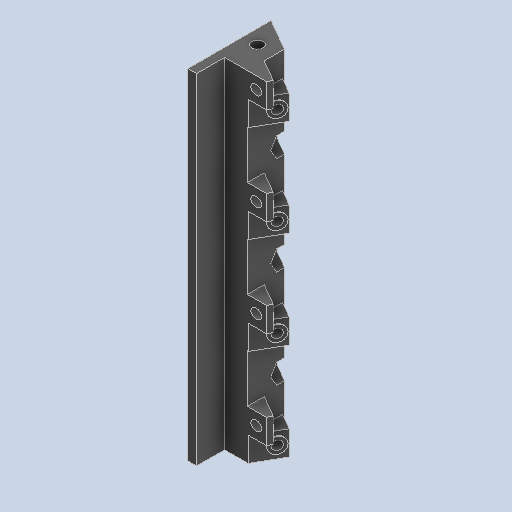
# Autodesk Inventor part: base_bearingpole_front
Saved by Autodesk Inventor 2024.1 (Build 281209000, 209)
## iProperties
Created: 2025-01-17
Part Number: base_bearingpole_front
Material: 一般
Document SubType Name: Modeling
Designer: hibik
Density: 1 g/cm^3
Appearance: 既定
Author: hibik
Autodesk Inventor part; units mm, degrees
ref_plane "YZ Plane" through (0, 0, 0) normal (1, 0, 0) x (0, 1, 0)
ref_plane "XZ Plane" through (0, 0, 0) normal (0, 1, 0) x (-1, 0, 0)
ref_plane "XY Plane" through (0, 0, 0) normal (0, 0, 1) x (1, 0, 0)
sketch "スケッチ1" plane through (0, 0, 0) normal (0, 1, 0) x (-1, 0, 0)
  line L0 (0, 0) -> (10, 0)
  line L1 (10, 0) -> (10, -23.7735)
  line L2 (0, 0) -> (0, -18) construction
  line L3 (0, -18) -> (10, -23.7735)
  line L4 (1, -18.5774) -> (1, 0)
  line L5 (-5, 0) -> (-5, -8)
  line L6 (0, -18) -> (-8.0801, -13.3349)
  line L7 (-8.0801, -13.3349) -> (-5, -8)
  line L8 (1, -12.8038) -> (-5.5801, -9.0048)
  line L9 (-1.25, -11.5048) -> (-3.75, -15.8349)
  line L10 (-5, -8) -> (1, -8)
  line L11 (-5.1471, -9.2548) -> (-4.4226, -8)
  line L12 (-1.25, -11.5048) -> (0.7735, -8)
  line L13 (-7.8301, -12.9019) -> (1, -18)
  line L14 (1, -8) -> (2, -8)
  line L15 (2, -8) -> (2, 0)
  line L16 (2, 0) -> (1, 0)
  line L17 (1, 0) -> (1, -8)
  point P0 (-3.5, -15.4019)
  dimension "d0" = 18
  dimension "d1" = 10
  dimension "d2" = 60
  dimension "d3" = 1
  dimension "d6" = 8
  dimension "d7" = 5
  dimension "d8" = 5
  dimension "d9" = 5
  dimension "d10" = 0.5
  dimension "d35" = 0.5
  dimension "d38" = 1
  constraints: 36 end point, 14 point on line, 5 perpendicular, 4 parallel, 4 vertical, 2 collinear, 2 horizontal
  measures "d0" distance of L0.start L2.end
  measures "d1" distance of L0.start L0.end
  measures "d2" angle of L2 L3
  measures "d3" distance between parallel lines of L2 L4
  measures "d6" distance of L5.start L5.end
  measures "d7" distance between parallel lines of L2 L5
  measures "d8" distance between parallel lines of L6 L8
  measures "d9" distance between parallel lines of L7 L9
  measures "d10" distance between parallel lines of L7 L11
  measures "d35" distance between parallel lines of L6 L13
  measures "d38" distance of L10.end L14.end
extrude "押し出し1" add sketch "スケッチ1" along normal blind 97 contours L0 L1 L3 L4 L14 L15
extrude "押し出し2" add sketch "スケッチ1" along normal blind 7 contours L4 L8 L12 L10 | L4 L13 L9 L8
sketch "スケッチ2" plane through (0, 7, 0) normal (0, 1, 0) x (1, 0, 0)
  line L0 (-1, 12.8038) -> (5.5801, 9.0048) projected
  line L1 (5.1471, 9.2548) -> (4.4226, 8) projected
  line L2 (5, 8) -> (-1, 8) projected
  line L3 (-1, 8) -> (-1, 18) projected
  point P0 (0, 0)
  point P1 (-1, 18.5774)
extrude "押し出し3" add sketch "スケッチ2" along normal blind 7
sketch "スケッチ3" plane through (3.75, 0, -15.8349) normal (0.8660254, 0, 0.5) x (0.5, 0, -0.8660254)
  circle A0 centre (-3, 3.5) radius 3
  line L0 (0, 0) -> (0, 7)
  circle A1 centre (-3, 3.5) radius 1.3
  line L1 (-0.5, 0) -> (-0.5, 7) projected
  point P0 (-15.5885, 0)
  point P1 (0, 3.5)
  dimension "d15" = 6
  dimension "d16" = 2.6
  dimension "d36" = 0.5
  constraints: 3 horizontal alignment, 2 centre point, 2 end point, 1 coincident, 1 midpoint, 1 tangent
  measures "d15" diameter of A0
  measures "d16" diameter of A1
  measures "d36" distance between parallel lines of L0 L1
extrude "押し出し4" cut sketch "スケッチ3" against normal blind 5 contours A1
sketch "スケッチ4" plane through (-1, 7, -12.8038) normal (0.5, 0, -0.8660254) x (-0.8660254, 0, -0.5)
  circle A0 centre (-4.5981, 3.5) radius 3
  line L0 (-7.5981, 0) -> (-7.5981, 7)
  circle A1 centre (-4.5981, 3.5) radius 1.35
  line L1 (-7.0981, 0) -> (-7.0981, 7) projected
  point P0 (-7.2679, -7)
  point P1 (-7.5981, 3.5)
  dimension "d19" = 6
  dimension "d20" = 2.7
  dimension "d37" = 0.5
  constraints: 3 horizontal alignment, 2 centre point, 2 end point, 1 coincident, 1 midpoint, 1 tangent
  measures "d19" diameter of A0
  measures "d20" diameter of A1
  measures "d37" distance between parallel lines of L1 L0
extrude "押し出し5" cut sketch "スケッチ4" against normal up to surface contours A1 surface through (-2, 0, -8) normal (0, 0, 1)
sketch "スケッチ5" plane through (3.75, 0, -15.8349) normal (0.8660254, 0, 0.5) x (0.5, 0, -0.8660254)
  circle A0 centre (-3, 3.5) radius 1.3 projected
  line L0 (-9.047, 0) -> (-0.5, 0) projected
  line L1 (-5, 7) -> (-0.5, 7) projected
  line L2 (-9.047, 7) -> (-5, 7) projected
  line L3 (-9.047, 0) -> (-9.047, 7) projected
  circle A1 centre (-3, 3.5) radius 2.25
  line L4 (-0.5, 0) -> (-0.5, 7) projected
  point P0 (-15.5885, 0)
  dimension "d26" = 4.5
  constraints: 1 centre point, 1 coincident
  measures "d26" diameter of A1
extrude "押し出し6" add sketch "スケッチ5" along normal blind 0.2 contours A1
sketch "スケッチ6" plane through (-1, 7, -12.8038) normal (0.5, 0, -0.8660254) x (-0.8660254, 0, -0.5)
  circle A0 centre (-4.5981, 3.5) radius 1.35 projected
  line L0 (-7.0981, 0) -> (-2.5981, 0) projected
  line L1 (0, 0) -> (-2.5981, 0) projected
  line L2 (0, 7) -> (0, 0) projected
  line L3 (-7.0981, 7) -> (0, 7) projected
  line L4 (-7.0981, 0) -> (-7.0981, 7) projected
  circle A1 centre (-4.5981, 3.5) radius 2.25
  point P0 (-7.2679, -7)
  dimension "d29" = 4.5
  constraints: 1 centre point, 1 coincident
  measures "d29" diameter of A1
extrude "押し出し7" add sketch "スケッチ6" along normal blind 0.2 contours A1
pattern_linear "矩形状パターン2" count 4 spacing 27.6667 along (0, 1, 0) of "押し出し2", "押し出し3", "押し出し4", "押し出し5", "押し出し6", "押し出し7"
sketch "スケッチ7" plane through (0, 97, 0) normal (0, 1, 0) x (1, 0, 0)
  line L0 (-8.85, 6.6454) -> (-6, 8.2909)
  line L1 (-6, 8.2909) -> (-3.15, 6.6454)
  line L2 (-3.15, 6.6454) -> (-3.15, 3.3546)
  line L3 (-3.15, 3.3546) -> (-6, 1.7091)
  line L4 (-6, 1.7091) -> (-8.85, 3.3546)
  line L5 (-8.85, 3.3546) -> (-8.85, 6.6454)
  line L6 (-8.85, 14.2184) -> (-8.85, 17.5093)
  line L7 (-8.85, 17.5093) -> (-6, 19.1547)
  line L8 (-6, 19.1547) -> (-3.15, 17.5093)
  line L9 (-3.15, 17.5093) -> (-3.15, 14.2184)
  line L10 (-3.15, 14.2184) -> (-6, 12.5729)
  line L11 (-6, 12.5729) -> (-8.85, 14.2184)
  line L12 (-10, 0) -> (-2, 0) projected
  line L13 (-10, 0) -> (-10, 23.7735) projected
  line L14 (-6, 19.1547) -> (-10, 19.1547)
  line L15 (-6, 12.5729) -> (-10, 12.5729)
  line L16 (-6, 8.2909) -> (-10, 8.2909)
  line L17 (-6, 1.7091) -> (-10, 1.7091)
  line L18 (-1, 18.5774) -> (-10, 23.7735) projected
  circle A0 centre (-6, 15.8638) radius 1.6
  circle A1 centre (-6, 5) radius 1.6
  point P0 (0, 0)
  point P1 (-6, 0)
  dimension "d39" = 5.7
  dimension "d40" = 5
  dimension "d41" = 2
  dimension "d42" = 3.2
  dimension "d43" = 3.2
  constraints: 32 end point, 4 perpendicular, 4 point on line, 2 centre point, 2 coincident, 2 vertical, 2 vertical alignment, 1 collinear, 1 midpoint, 26 other
  measures "d39" distance between parallel lines of L5 L2
  measures "d40" distance from line of L12 point (-6, 5)
  measures "d41" distance between parallel lines of L18 L8
  measures "d42" diameter of A0
  measures "d43" diameter of A1
extrude "押し出し8" cut sketch "スケッチ7" against normal blind 15 contours A0
sketch "スケッチ9" plane through (0, 97, 0) normal (0, 1, 0) x (1, 0, 0)
  circle A0 centre (-6, 15.8638) radius 1.6 projected
  line L0 (-10, 23.7735) -> (-10, 0) projected
  line L1 (-10, 23.7735) -> (-10, 0) projected
  line L2 (-8.85, 14.2184) -> (-8.85, 17.5093)
  line L3 (-8.85, 17.5093) -> (-6, 19.1547)
  line L4 (-6, 19.1547) -> (-3.15, 17.5093)
  line L5 (-3.15, 17.5093) -> (-3.15, 14.2184)
  line L6 (-3.15, 14.2184) -> (-6, 12.5729)
  line L7 (-6, 12.5729) -> (-8.85, 14.2184)
  line L8 (-3.15, 3.3546) -> (-6, 1.7091)
  line L9 (-6, 1.7091) -> (-8.85, 3.3546)
  line L10 (-8.85, 3.3546) -> (-8.85, 6.6454)
  line L11 (-8.85, 6.6454) -> (-6, 8.2909)
  line L12 (-6, 8.2909) -> (-3.15, 6.6454)
  line L13 (-3.15, 6.6454) -> (-3.15, 3.3546)
  line L14 (-6, 19.1547) -> (-10, 19.1547)
  line L15 (-6, 12.5729) -> (-10, 12.5729)
  line L16 (-6, 8.2909) -> (-10, 8.2909)
  line L17 (-6, 1.7091) -> (-10, 1.7091)
  point P0 (0, 0)
  point P1 (-6, 5)
  point P2 (-6, 5)
  dimension "d46" = 5.7
  constraints: 32 end point, 4 perpendicular, 4 point on line, 2 coincident, 2 collinear, 26 other
  measures "d46" distance between parallel lines of L10 L13
extrude "押し出し9" cut sketch "スケッチ9" against normal blind 6 contours L14 L3 L2 L7 L15 L0 | L4 L5 L6 L7 L2 L3
extrude "押し出し10" add sketch "スケッチ9" against normal blind 3 contours L14 L3 L2 L7 L15 L0 | L4 L5 L6 L7 L2 L3
ref_plane "作業平面1" through (0, 48.5, 0) normal (0, 1, 0) x (1, 0, 0)
mirror "ミラー1" about plane through (0, 48.5, 0) normal (0, 1, 0) of "押し出し9", "押し出し10", "押し出し8"
sketch "スケッチ10" plane through (-1, 0, -18.5774) normal (1, 0, 0) x (0, 0, -1)
  line L0 (2.7135, 17.85) -> (1.0681, 15)
  line L1 (1.0681, 15) -> (-2.2228, 15)
  line L2 (-2.2228, 15) -> (-3.8682, 17.85)
  line L3 (-3.8682, 17.85) -> (-2.2228, 20.7)
  line L4 (-2.2228, 20.7) -> (1.0681, 20.7)
  line L5 (1.0681, 20.7) -> (2.7135, 17.85)
  line L6 (-18.5774, 0) -> (-10.5774, 0) projected
  circle A0 centre (-0.5774, 17.85) radius 1.6
  line L7 (-18.5774, 0) -> (-18.5774, 97) projected
  line L8 (1.0681, 20.7) -> (5.1962, 20.7)
  line L9 (5.1962, 20.7) -> (5.1962, 15)
  line L10 (5.1962, 15) -> (1.0681, 15)
  line L11 (5.1962, 0) -> (5.1962, 97) projected
  point P0 (-14.5774, 0)
  dimension "d52" = 5.7
  dimension "d53" = 15
  dimension "d54" = 3.2
  dimension "d64" = 18
  constraints: 18 end point, 2 horizontal, 2 perpendicular, 1 centre point, 1 coincident, 1 collinear, 1 midpoint, 13 other
  measures "d52" distance between parallel lines of L1 L4
  measures "d53" distance from line of point (-14.577, 0) L1
  measures "d54" diameter of A0
  measures "d64" distance from line of L7 point (-0.577, 17.85)
extrude "押し出し11" cut sketch "スケッチ10" against normal blind 5 contours L5 L8 L9 L10 L0 | L0 L1 L2 L3 L4 L5 | A0
extrude "押し出し12" cut sketch "スケッチ10" against normal through all contours A0
pattern_linear "矩形状パターン3" count 3 spacing 28 along (0, 1, 0) of "押し出し11", "押し出し12"
sketch "スケッチ12" plane through (0, 97, 0) normal (0, 1, 0) x (1, 0, 0)
  line L0 (-2, 0) -> (-2, 8) projected
  line L1 (-2, 8) -> (-7.5, 8)
  line L2 (-7.5, 8) -> (-7.5, 0)
  line L3 (-7.5, 0) -> (-2, 0)
  line L4 (-2, 0) -> (-2, 8)
  line L5 (-10, 0) -> (-2, 0) projected
  line L6 (-10, 23.7735) -> (-10, 0) projected
  point P0 (0, 0)
  dimension "d65" = 2.5
  dimension "d68" = 8
  constraints: 8 end point, 2 parallel, 1 collinear, 1 horizontal, 1 perpendicular
  measures "d65" distance between parallel lines of L6 L2
  measures "d68" distance of L0.start L0.end
extrude "押し出し14" cut sketch "スケッチ12" against normal through all
